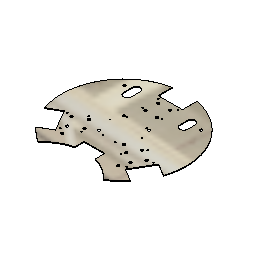
BaseChapaMeio (Autodesk Fusion 360 design; units mm, degrees)
Autodesk Fusion 360 part; units mm, degrees
note: some values were not read from the file. Set by a fixed rule: which sketch regions a step uses.
sketch "Sketch1" plane through (0, 0, 0) normal (0, 1, 0) x (1, 0, 0)
  circle A0 centre (0, 0) radius 240
  line L0 (0, -240) -> (125, -240)
  line L1 (125, -240) -> (125, -204.878)
  line L2 (0, 240) -> (0, -147)
  line L3 (125, -204.878) -> (-125, -204.878)
  arc A1 (125, -204.878) -> (-125, -204.878) centre (0, -310.9212) ccw
  circle A2 centre (-53.8749, 53.8749) radius 5
  line L4 (-53.8749, 53.8749) -> (51.1251, 53.8749)
  line L5 (51.1251, 53.8749) -> (51.1251, -51.1251)
  line L6 (51.1251, -51.1251) -> (-53.8749, -51.1251)
  line L7 (-53.8749, -51.1251) -> (-53.8749, 53.8749)
  circle A3 centre (51.1251, 53.8749) radius 5
  circle A4 centre (51.1251, -51.1251) radius 5
  circle A5 centre (-53.8749, -51.1251) radius 5
  line L8 (0, 240) -> (250, 240)
  line L9 (-53.8749, 53.8749) -> (-53.8749, 233.8749)
  line L10 (-53.8749, 53.8749) -> (-233.8749, 53.8749)
  line L11 (0, -147) -> (40, -147)
  line L12 (40, -147) -> (40, -151.9553)
  line L13 (0, -147) -> (0, -95)
  line L14 (0, -95) -> (-40, -95)
  line L15 (40, -151.9553) -> (-40, -151.9553)
  line L16 (-40, -151.9553) -> (-40, -95)
  line L17 (-40, -95) -> (40, -95)
  line L18 (40, -95) -> (40, -151.9553)
  line L19 (0, 0) -> (207.8461, -120)
  line L20 (0, 0) -> (240, 0) construction
  line L21 (0, 0) -> (-207.8461, -120)
  line L22 (0, 0) -> (0, 240)
  line L23 (0, 240) -> (45, 240)
  line L24 (45, 240) -> (-45, 240)
  line L25 (-45, 240) -> (-45, 187)
  line L26 (-45, 187) -> (45, 187)
  line L27 (45, 187) -> (45, 240)
  line L28 (207.8461, -120) -> (185.3461, -158.9711)
  line L29 (207.8461, -120) -> (230.3461, -81.0289)
  line L30 (230.3461, -81.0289) -> (184.4468, -54.5289)
  line L31 (184.4468, -54.5289) -> (139.4468, -132.4711)
  line L32 (139.4468, -132.4711) -> (185.3461, -158.9711)
  line L33 (-207.8461, -120) -> (-185.3461, -158.9711)
  line L34 (-185.3461, -158.9711) -> (-139.4468, -132.4711)
  line L35 (-139.4468, -132.4711) -> (-184.4468, -54.5289)
  line L36 (-184.4468, -54.5289) -> (-230.3461, -81.0289)
  line L37 (-207.8461, -120) -> (-230.3461, -81.0289)
  line L38 (-40, -95) -> (-40, -75)
  line L39 (-40, -75) -> (40, -75)
  line L40 (40, -75) -> (40, 74)
  line L41 (40, 74) -> (-40, 74)
  line L42 (0, -75) -> (21, -75)
  line L43 (21, -75) -> (-21, -75)
  line L44 (-21, -75) -> (-21, 74)
  line L45 (21, -75) -> (21, 74)
  circle A6 centre (-21, 74) radius 2
  circle A7 centre (21, 74) radius 2
  circle A8 centre (-21, -75) radius 2
  circle A9 centre (21, -75) radius 2
  line L46 (-139.4468, -132.4711) -> (-143.4468, -125.5429)
  line L47 (-184.4468, -54.5289) -> (-180.4468, -61.4571)
  line L48 (-143.4468, -125.5429) -> (-134.7865, -120.5429)
  line L49 (-134.7865, -120.5429) -> (-82.825, -90.5429)
  line L50 (-82.825, -90.5429) -> (-22.2032, -55.5429)
  line L51 (-139.4468, -132.4711) -> (-151.9468, -110.8205)
  line L52 (-151.9468, -110.8205) -> (-130.2961, -98.3205)
  line L53 (-130.2961, -98.3205) -> (-86.9948, -73.3205)
  line L54 (-184.4468, -54.5289) -> (-171.9468, -76.1795)
  line L55 (-171.9468, -76.1795) -> (-150.2961, -63.6795)
  line L56 (-150.2961, -63.6795) -> (-106.9948, -38.6795)
  line L57 (-180.4468, -61.4571) -> (-171.7865, -56.4571)
  line L58 (-171.7865, -56.4571) -> (-119.825, -26.4571)
  line L59 (-119.825, -26.4571) -> (-59.2032, 8.5429)
  circle A10 centre (-22.2032, -55.5429) radius 2.5
  circle A11 centre (-82.825, -90.5429) radius 2.5
  circle A12 centre (-134.7865, -120.5429) radius 2.5
  circle A13 centre (-59.2032, 8.5429) radius 2.5
  circle A14 centre (-119.825, -26.4571) radius 2.5
  circle A15 centre (-171.7865, -56.4571) radius 2.5
  circle A16 centre (-106.9948, -38.6795) radius 2.5
  circle A17 centre (-150.2961, -63.6795) radius 2.5
  circle A18 centre (-86.9948, -73.3205) radius 2.5
  circle A19 centre (-130.2961, -98.3205) radius 2.5
  circle A20 centre (59.2032, 8.5429) radius 2.5
  circle A21 centre (119.825, -26.4571) radius 2.5
  circle A22 centre (171.7865, -56.4571) radius 2.5
  circle A23 centre (150.2961, -63.6795) radius 2.5
  line L60 (150.2961, -63.6795) -> (106.9948, -38.6795)
  circle A24 centre (106.9948, -38.6795) radius 2.5
  circle A25 centre (130.2961, -98.3205) radius 2.5
  circle A26 centre (86.9948, -73.3205) radius 2.5
  circle A27 centre (82.825, -90.5429) radius 2.5
  circle A28 centre (134.7865, -120.5429) radius 2.5
  circle A29 centre (22.2032, -55.5429) radius 2.5
  line L61 (82.825, -90.5429) -> (22.2032, -55.5429)
  line L62 (134.7865, -120.5429) -> (82.825, -90.5429)
  line L63 (143.4468, -125.5429) -> (134.7865, -120.5429)
  line L64 (151.9468, -110.8205) -> (130.2961, -98.3205)
  line L65 (130.2961, -98.3205) -> (86.9948, -73.3205)
  line L66 (171.9468, -76.1795) -> (150.2961, -63.6795)
  line L67 (180.4468, -61.4571) -> (171.7865, -56.4571)
  line L68 (171.7865, -56.4571) -> (119.825, -26.4571)
  line L69 (119.825, -26.4571) -> (59.2032, 8.5429)
  circle A30 centre (-37, 47) radius 2.5
  circle A31 centre (-37, 117) radius 2.5
  circle A32 centre (-37, 177) radius 2.5
  circle A33 centre (-20, 162) radius 2.5
  line L70 (-20, 162) -> (-20, 112)
  circle A34 centre (-20, 112) radius 2.5
  circle A35 centre (20, 162) radius 2.5
  circle A36 centre (20, 112) radius 2.5
  circle A37 centre (37, 117) radius 2.5
  circle A38 centre (37, 177) radius 2.5
  circle A39 centre (37, 47) radius 2.5
  line L71 (37, 117) -> (37, 47)
  line L72 (37, 177) -> (37, 117)
  line L73 (37, 187) -> (37, 177)
  line L74 (20, 187) -> (20, 162)
  line L75 (20, 162) -> (20, 112)
  line L76 (-20, 187) -> (-20, 162)
  line L77 (-37, 187) -> (-37, 177)
  line L78 (-37, 177) -> (-37, 117)
  line L79 (-37, 117) -> (-37, 47)
  circle A40 centre (120.8737, -122.997) radius 5
  circle A41 centre (-120.8737, -122.997) radius 5
  line L80 (147.6404, 0) -> (147.6404, 146)
  circle A42 centre (147.6404, 146) radius 5
  line L81 (147.6404, 146) -> (106.1404, 146)
  line L82 (106.1404, 146) -> (106.1404, 169)
  line L83 (106.1404, 146) -> (106.1404, 129)
  line L84 (92.1404, 169) -> (92.1404, 129)
  arc A43 (92.1404, 129) -> (120.1404, 129) centre (106.1404, 129) ccw
  line L85 (120.1404, 129) -> (120.1404, 169)
  arc A44 (120.1404, 169) -> (92.1404, 169) centre (106.1404, 169) ccw
  line L86 (106.1404, 169) -> (106.1404, 129) construction
  line L87 (106.1404, 169) -> (-103.8596, 169)
  line L88 (106.1404, 129) -> (-103.8596, 129)
  line L89 (147.6404, 146) -> (-149.3596, 146)
  circle A45 centre (-149.3596, 146) radius 5
  line L90 (-117.8596, 169) -> (-117.8596, 129)
  arc A46 (-117.8596, 129) -> (-89.8596, 129) centre (-103.8596, 129) ccw
  line L91 (-89.8596, 129) -> (-89.8596, 169)
  arc A47 (-89.8596, 169) -> (-117.8596, 169) centre (-103.8596, 169) ccw
  line L92 (-103.8596, 169) -> (-103.8596, 129) construction
  point P0 (-106.9948, -38.6795)
  point P1 (-150.2961, -63.6795)
  point P2 (-59.2032, 8.5429)
  point P3 (-119.825, -26.4571)
  point P4 (-171.7865, -56.4571)
  dimension "d2" = 125
  dimension "d3" = 387
  dimension "d7" = 10
  dimension "d8" = 105
  dimension "d9" = 105
  dimension "d10" = 10
  dimension "d11" = 10
  dimension "d12" = 10
  dimension "d13" = 250
  dimension "d14" = 180
  dimension "d15" = 180
  dimension "d22" = 40
  dimension "d23" = 52
  dimension "d24" = 40
  dimension "d40" = 30
  dimension "d41" = 60
  dimension "d42" = 240
  dimension "d46" = 45
  dimension "d47" = 90
  dimension "d48" = 53
  dimension "d49" = 45
  dimension "d50" = 45
  dimension "d53" = 45
  dimension "d54" = 53
  dimension "d55" = 90
  dimension "d56" = 53
  dimension "d57" = 20
  dimension "d58" = 80
  dimension "d59" = 149
  dimension "d60" = 80
  dimension "d61" = 21
  dimension "d62" = 42
  dimension "d63" = 4
  dimension "d64" = 4
  dimension "d65" = 4
  dimension "d66" = 4
  dimension "d67" = 8
  dimension "d68" = 8
  dimension "d69" = 10
  dimension "d70" = 60
  dimension "d71" = 70
  dimension "d72" = 25
  dimension "d73" = 25
  dimension "d74" = 50
  dimension "d75" = 25
  dimension "d76" = 5
  dimension "d77" = 5
  dimension "d78" = 5
  dimension "d79" = 5
  dimension "d80" = 5
  dimension "d81" = 5
  dimension "d82" = 5
  dimension "d83" = 5
  dimension "d84" = 5
  dimension "d85" = 5
  dimension "d87" = 360
  dimension "d33" = 10
  dimension "d89" = 146
  dimension "d90" = 10
  dimension "d91" = 41.5
  dimension "d92" = 23
  dimension "d93" = 17
  dimension "d94" = 28
  dimension "d95" = 210
  dimension "d96" = 210
  dimension "d97" = 297
  dimension "d98" = 10
  dimension "d99" = 28
  constraint coincident A0.centre L19.start
  constraint coincident A0 L0.start
  constraint horizontal L0
  constraint coincident A0 L1.end
  constraint perpendicular L0 L1
  constraint coincident A0 L2.start
  constraint vertical L2
  constraint coincident A0 L3.end
  constraint perpendicular L1 L3
  constraint coincident L2.end A1
  constraint horizontal L4
  constraint vertical L5
  constraint horizontal L6
  constraint vertical L7
  constraint coincident A2.centre L4.start
  constraint coincident L4.end L5.start
  constraint coincident L5.end L6.start
  constraint coincident L6.end L7.start
  constraint perpendicular L2 L8
  constraint coincident A0 L9.end
  constraint parallel L7 L9
  constraint coincident A0 L10.end
  constraint perpendicular L9 L10
  constraint perpendicular L2 L11
  constraint coincident A1 L12.end
  constraint perpendicular L11 L12
  constraint perpendicular L11 L13
  constraint perpendicular L2 L14
  constraint horizontal L15
  constraint vertical L16
  constraint horizontal L17
  constraint vertical L18
  constraint horizontal L20
  constraint perpendicular L2 L23
  constraint horizontal L24
  constraint vertical L25
  constraint horizontal L26
  constraint vertical L27
  constraint perpendicular L19 L28
  constraint perpendicular L19 L29
  constraint perpendicular L29 L30
  constraint perpendicular L30 L31
  constraint perpendicular L21 L33
  constraint perpendicular L33 L34
  constraint perpendicular L34 L35
  constraint perpendicular L35 L36
  constraint perpendicular L17 L38
  constraint perpendicular L16 L39
  constraint perpendicular L6 L40
  constraint perpendicular L40 L41
  constraint midpoint L39 L42.start
  constraint perpendicular L2 L42
  constraint parallel L39 L43
  constraint coincident L41 L44.end
  constraint perpendicular L41 L44
  constraint coincident L41 L45.end
  constraint perpendicular L41 L45
  constraint coincident L44.end A6.centre
  constraint coincident L45.end A7.centre
  constraint coincident L43.end L44.start
  constraint coincident L42.end L43.start
  constraint perpendicular L34 L46
  constraint perpendicular L36 L47
  constraint perpendicular L46 L48
  constraint parallel L48 L49
  constraint parallel L49 L50
  constraint perpendicular L48 L51
  constraint perpendicular L51 L52
  constraint parallel L52 L53
  constraint symmetric L21 L52.end P1
  constraint symmetric L21 L53.end P0
  constraint perpendicular L36 L54
  constraint coincident P1 L55.end
  constraint coincident P0 L56.end
  constraint symmetric L21 L48.end P4
  constraint symmetric L21 L49.end P3
  constraint symmetric L21 L50.end P2
  constraint coincident P4 L57.end
  constraint coincident P3 L58.end
  constraint coincident P2 L59.end
  constraint coincident L50.end A10.centre
  constraint coincident L49.end L50.start
  constraint coincident L48.end L49.start
  constraint coincident L53.end A18.centre
  constraint coincident L52.end L53.start
  constraint coincident L20 L80.start
  constraint coincident L80.end A42.centre
  constraint perpendicular L80 L81
  constraint perpendicular L81 L82
  constraint perpendicular L81 L83
  constraint tangent L84 A43
  constraint tangent A43 L85
  constraint parallel L84 L85
  constraint tangent L85 A44
  constraint tangent L84 A44
  constraint coincident L83.end A43.centre
  constraint parallel L83 L86
  constraint coincident L82.end A44.centre
  constraint perpendicular L86 L87
  constraint perpendicular L9 L88
  constraint perpendicular L86 L89
  constraint coincident L89.end A45.centre
  constraint tangent L90 A46
  constraint tangent A46 L91
  constraint parallel L90 L91
  constraint tangent L91 A47
  constraint tangent L90 A47
  constraint coincident L88.end A46.centre
  constraint perpendicular L88 L92
  constraint coincident L87.end A47.centre
  measures "d2" distance of L0.start L0.end
  measures "d3" distance of L2.start L2.end
  measures "d7" diameter of A2
  measures "d8" distance of A2.centre L4.end
  measures "d9" distance of A2.centre L6.end
  measures "d10" diameter of A3
  measures "d11" diameter of A4
  measures "d12" diameter of A5
  measures "d13" distance of L2.start L8.end
  measures "d14" distance of A2.centre L10.end
  measures "d15" distance of A2.centre L9.end
  measures "d22" distance of L2.end L11.end
  measures "d23" distance of L2.end L13.end
  measures "d24" distance of L13.end L14.end
  measures "d40" angle of L19 L20
  measures "d41" angle of L19 L21
  measures "d42" distance of A0.centre L21.end
  measures "d46" distance of L2.start L23.end
  measures "d47" distance of L23.end L24.end
  measures "d48" distance of L23.end L26.end
  measures "d49" distance of L19.end L28.end
  measures "d50" distance of L19.end L29.end
  measures "d53" distance of L21.end L33.end
  measures "d54" distance of L33.end L34.end
  measures "d55" distance of L34.end L35.end
  measures "d56" distance of L35.end L36.end
  measures "d57" distance of L14.end L38.end
  measures "d58" distance of L38.end L39.end
  measures "d59" distance of L39.end L40.end
  measures "d60" distance of L40.end L41.end
  measures "d61" distance of L42.start L42.end
  measures "d62" distance of L42.end L43.end
  measures "d63" diameter of A6
  measures "d64" diameter of A7
  measures "d65" diameter of A8
  measures "d66" diameter of A9
  measures "d67" distance of L34.end L46.end
  measures "d68" distance of L35.end L47.end
  measures "d69" distance of L46.end L48.end
  measures "d70" distance of L48.end L49.end
  measures "d71" distance of L49.end L50.end
  measures "d72" distance of L34.end L51.end
  measures "d73" distance of L51.end L52.end
  measures "d74" distance of L52.end L53.end
  measures "d75" distance of L35.end L54.end
  measures "d76" diameter of A10
  measures "d77" diameter of A11
  measures "d78" diameter of A12
  measures "d79" diameter of A13
  measures "d80" diameter of A14
  measures "d81" diameter of A15
  measures "d82" diameter of A16
  measures "d83" diameter of A17
  measures "d84" diameter of A18
  measures "d85" diameter of A19
  measures "d33" diameter of A41
  measures "d89" distance of L80.start L80.end
  measures "d90" diameter of A42
  measures "d91" distance of L80.end L81.end
  measures "d92" distance of L81.end L82.end
  measures "d93" distance of L81.end L83.end
  measures "d94" diameter of A43
  measures "d95" distance of L82.end L87.end
  measures "d96" distance of L83.end L88.end
  measures "d97" distance of L80.end L89.end
  measures "d98" diameter of A45
  measures "d99" diameter of A46
sketch "Sketch2" plane through (0, 0, 0) normal (0, 1, 0) x (1, 0, 0)
  circle A0 centre (0, 0) radius 240
  line L0 (0, 0) -> (0, 240)
  line L1 (0, 240) -> (0, 180)
  line L2 (0, 180) -> (45, 180)
  line L3 (45, 180) -> (45, 235.7435)
  line L4 (0, 180) -> (-3.838, 180)
  line L5 (-3.838, 180) -> (-48.838, 180)
  line L6 (-48.838, 180) -> (-48.838, 234.9784)
  circle A1 centre (-24.1183, -57.226) radius 2.5
  line L7 (-37.5, 180) -> (-37.5, 169.5)
  circle A2 centre (-113.5798, -22.274) radius 2.5
  circle A3 centre (-37.5, 109.5) radius 2.5
  circle A4 centre (-128.0413, -117.226) radius 2.5
  line L8 (0, 0) -> (0, 240)
  circle A5 centre (165.5413, -52.274) radius 2.5
  circle A6 centre (76.0798, -87.226) radius 2.5
  line L9 (37.5, 169.5) -> (37.5, 109.5)
  line L10 (0, 240) -> (0, 180)
  circle A7 centre (37.5, 109.5) radius 2.5
  line L11 (0, 0) -> (207.8461, -120)
  circle A8 centre (37.5, 49.5) radius 2.5
  line L12 (45, 180) -> (45, 235.7435)
  circle A9 centre (113.5798, -22.274) radius 2.5
  circle A10 centre (0, 0) radius 240
  line L13 (0, 180) -> (45, 180)
  circle A11 centre (37.5, 169.5) radius 2.5
  line L14 (37.5, 180) -> (37.5, 169.5)
  line L15 (37.5, 109.5) -> (37.5, 49.5)
  line L16 (0, 0) -> (240, 0) construction
  line L17 (0, 180) -> (-45, 180)
  line L18 (0, 180) -> (-37.5, 180)
  circle A12 centre (-61.6183, 7.726) radius 2.5
  line L19 (0, 0) -> (-207.8461, -120)
  circle A13 centre (61.6183, 7.726) radius 2.5
  circle A14 centre (-37.5, 169.5) radius 2.5
  circle A15 centre (-76.0798, -87.226) radius 2.5
  circle A16 centre (-37.5, 49.5) radius 2.5
  circle A17 centre (-165.5413, -52.274) radius 2.5
  line L20 (-37.5, 109.5) -> (-37.5, 49.5)
  line L21 (-37.5, 169.5) -> (-37.5, 109.5)
  circle A18 centre (24.1183, -57.226) radius 2.5
  line L22 (0, 0) -> (240, 0) construction
  circle A19 centre (128.0413, -117.226) radius 2.5
  line L23 (0, 180) -> (22.5, 180)
  line L24 (22.5, 180) -> (22.5, 154)
  line L25 (22.5, 154) -> (22.5, 105)
  circle A20 centre (22.5, 154) radius 5
  circle A21 centre (22.5, 105) radius 5
  circle A22 centre (-22.5, 105) radius 5
  circle A23 centre (-22.5, 154) radius 5
  circle A24 centre (-144.6179, -57.5144) radius 5
  circle A25 centre (-122.1179, -96.4856) radius 5
  circle A26 centre (-128.0413, -117.226) radius 2.5
  circle A27 centre (-76.0798, -87.226) radius 2.5
  circle A28 centre (-79.6827, -71.9856) radius 5
  circle A29 centre (-102.1827, -33.0144) radius 5
  circle A30 centre (-113.5798, -22.274) radius 2.5
  circle A31 centre (-165.5413, -52.274) radius 2.5
  circle A32 centre (-24.1183, -57.226) radius 2.5
  circle A33 centre (-61.6183, 7.726) radius 2.5
  circle A34 centre (122.1179, -96.4856) radius 5
  circle A35 centre (144.6179, -57.5144) radius 5
  circle A36 centre (165.5413, -52.274) radius 2.5
  circle A37 centre (113.5798, -22.274) radius 2.5
  circle A38 centre (102.1827, -33.0144) radius 5
  circle A39 centre (79.6827, -71.9856) radius 5
  circle A40 centre (76.0798, -87.226) radius 2.5
  circle A41 centre (128.0413, -117.226) radius 2.5
  circle A42 centre (61.6183, 7.726) radius 2.5
  circle A43 centre (24.1183, -57.226) radius 2.5
  line L26 (-131.4656, -132.295) -> (-179.0783, -159.7842)
  line L27 (-178.3846, -51.0289) -> (-226.6599, -78.9006)
  line L28 (-155.8846, -90) -> (-178.3846, -51.0289)
  line L29 (-155.8846, -90) -> (-133.3846, -128.9711)
  line L30 (-153.9656, -93.3238) -> (-131.4656, -132.295)
  line L31 (180.3036, -47.705) -> (227.9163, -75.1942)
  line L32 (133.3846, -128.9711) -> (181.6599, -156.8429)
  line L33 (155.8846, -90) -> (133.3846, -128.9711)
  line L34 (155.8846, -90) -> (178.3846, -51.0289)
  line L35 (157.8036, -86.6762) -> (180.3036, -47.705)
  circle A44 centre (-107.5583, -130.5) radius 5
  circle A45 centre (107.9417, -130.5) radius 5
  circle A46 centre (149.1333, 148.0857) radius 5
  arc A47 (120.5391, 154.5493) -> (90.5391, 154.5493) centre (105.5391, 154.5493) ccw
  line L36 (120.5391, 124.5493) -> (120.5391, 154.5493)
  arc A48 (90.5391, 124.5493) -> (120.5391, 124.5493) centre (105.5391, 124.5493) ccw
  line L37 (90.5391, 154.5493) -> (90.5391, 124.5493)
  arc A49 (-95.8667, 159.0843) -> (-125.8667, 159.0843) centre (-110.8667, 159.0843) ccw
  line L38 (-95.8667, 124.0843) -> (-95.8667, 159.0843)
  arc A50 (-125.8667, 124.0843) -> (-95.8667, 124.0843) centre (-110.8667, 124.0843) ccw
  line L39 (-125.8667, 159.0843) -> (-125.8667, 124.0843)
  circle A51 centre (-145.8667, 148.0857) radius 5
  circle A52 centre (48.706, 47.294) radius 5
  circle A53 centre (-47.294, 47.294) radius 5
  circle A54 centre (-47.294, -48.706) radius 5
  circle A55 centre (48.706, -48.706) radius 5
  arc A56 (125.0048, -204.8751) -> (-125.0048, -204.8751) centre (0, -310.93) ccw
  line L40 (-38.4014, -152.3633) -> (-38.4014, -115.0053)
  line L41 (-38.4014, -115.0053) -> (41.5986, -115.0053)
  line L42 (41.5986, -115.0053) -> (41.5986, -152.3633)
  dimension "d100" = 480
  dimension "d101" = 60
  dimension "d102" = 45
  dimension "d103" = 45
  dimension "d107" = 360
  dimension "d108" = 480
  dimension "d109" = 150
  dimension "d110" = 30
  dimension "d111" = 60
  dimension "d112" = 45
  dimension "d113" = 45
  dimension "d114" = 37.5
  dimension "d115" = 10.5
  dimension "d116" = 5
  dimension "d117" = 60
  dimension "d118" = 60
  dimension "d119" = 5
  dimension "d120" = 5
  dimension "d123" = 22.5
  dimension "d124" = 26
  dimension "d125" = 49
  dimension "d126" = 10
  dimension "d127" = 10
  dimension "d129" = 360
  dimension "d131" = 360
  dimension "d132" = 10
  dimension "d133" = 10
  dimension "d134" = 10
  dimension "d135" = 10
  dimension "d21" = 30
  dimension "d27" = 10
  dimension "d30" = 30
  dimension "d139" = 10
  dimension "d140" = 10
  dimension "d43" = 10
  constraint coincident A0.centre L0.start
  constraint coincident A0 L0.end
  constraint vertical L0
  constraint parallel L0 L1
  constraint perpendicular L1 L2
  constraint coincident A0 L3.end
  constraint perpendicular L2 L3
  constraint perpendicular L1 L4
  constraint perpendicular L1 L5
  constraint coincident A0 L6.end
  constraint perpendicular L5 L6
  constraint horizontal L16
  constraint horizontal L22
  constraint coincident L0.end A10
  constraint perpendicular L8 L16
  constraint parallel L8 L10
  constraint perpendicular L10 L17
  constraint perpendicular L10 L13
  constraint coincident L3.end A10
  constraint perpendicular L12 L13
  constraint perpendicular L10 L18
  constraint perpendicular L7 L17
  constraint coincident L7.end A14.centre
  constraint parallel L7 L21
  constraint parallel L20 L21
  constraint coincident A3.centre L20.start
  constraint coincident A16.centre L20.end
  constraint symmetric L14.start L7.start L8
  constraint symmetric L9.start L7.end L8
  constraint symmetric L8 A11 A14
  constraint symmetric L7.end L9.start L8
  constraint symmetric A3.centre L9.end L8
  constraint symmetric A16.centre A8.centre L8
  constraint symmetric A3 L8 A7
  constraint symmetric L8 A8 A16
  constraint perpendicular L0 L23
  constraint perpendicular L2 L24
  constraint parallel L24 L25
  constraint coincident L24.end L25.start
  constraint coincident L25.end A21.centre
  constraint symmetric L8 A20 A23
  constraint symmetric L8 A21 A22
  constraint tangent A47 L36
  constraint tangent A47 L37
  constraint parallel L36 L37
  constraint tangent A48 L37
  constraint tangent L36 A48
  constraint tangent A50 L39
  constraint tangent L38 A50
  constraint parallel L38 L39
  constraint tangent A49 L38
  constraint tangent A49 L39
  constraint vertical L40
  constraint horizontal L41
  constraint vertical L42
  measures "d100" diameter of A0
  measures "d101" distance of L0.end L1.end
  measures "d102" distance of L1.end L2.end
  measures "d103" distance of L4.end L5.end
  measures "d108" diameter of A10
  measures "d109" angle of L16 L19
  measures "d110" angle of L11 L22
  measures "d111" distance of L1.end L0.end
  measures "d112" distance of L1.end L17.end
  measures "d113" distance of L1.end L2.end
  measures "d114" distance of L1.end L7.start
  measures "d115" distance of L7.start L7.end
  measures "d116" diameter of A14
  measures "d117" distance of A3.centre L7.end
  measures "d118" distance of A3.centre A16.centre
  measures "d119" diameter of A3
  measures "d120" diameter of A16
  measures "d123" distance of L1.end L23.end
  measures "d124" distance of L23.end L24.end
  measures "d125" distance of L24.end L25.end
  measures "d126" diameter of A20
  measures "d127" diameter of A21
  measures "d132" diameter of A53
  measures "d133" diameter of A52
  measures "d134" diameter of A55
  measures "d135" diameter of A54
  measures "d21" diameter of A47
  measures "d27" diameter of A51
  measures "d30" diameter of A50
  measures "d139" diameter of A44
  measures "d140" diameter of A45
  measures "d43" diameter of A46
extrude "Extrude2" add sketch "Sketch2" along normal blind 3 contours A0 L0 L2 L3 L8 L11 L12 A10 L13 L23 L31 L34 L35 | A0 L0 L4 L5 L6 L8 A10 L17 L18 L19 L27 L28 | A0 L11 A10 L19 L26 L29 L30 L32 L33 A56 L40 L41 L42
equation "d2 = ( 250 / 2 ) * 1 mm"
equation "d3 = 355 mm + 32 mm"
equation "d61 = ( 42 / 2 ) * 1 mm"
equation "d93 = 40 mm - 23 mm"
equation "d103 = ( 90 / 2 ) * 1 mm"
equation "d110 = 150 deg - 120 deg"
equation "d112 = ( 90 / 2 ) * 1 mm"
equation "d113 = ( 90 / 2 ) * 1 mm"
equation "d123 = ( 45 / 2 ) * 1 mm"
equation "d125 = 75 mm - 26 mm"
